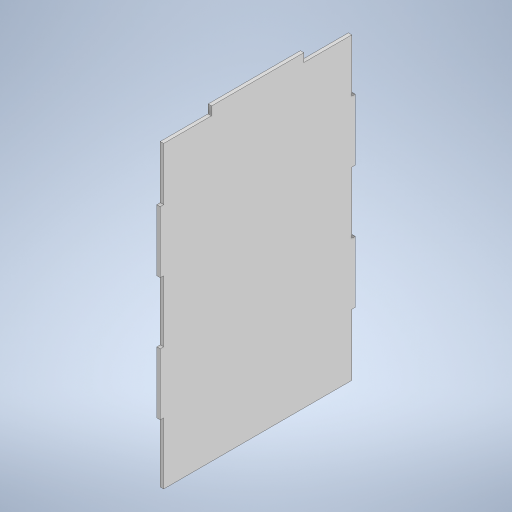
# Autodesk Inventor part: inner_side
Saved by Autodesk Inventor 2023 (Build 270158000, 158)
## iProperties
Created: 2023-04-26
Part Number: inner_side
Material: Generic
Document SubType Name: Modeling
Designer: Unnar
Density: 1 g/cm^3
Appearance: Default
Author: Unnar
Autodesk Inventor part; units mm, degrees
ref_plane "YZ Plane" through (0, 0, 0) normal (1, 0, 0) x (0, 1, 0)
ref_plane "XZ Plane" through (0, 0, 0) normal (0, 1, 0) x (-1, 0, 0)
ref_plane "XY Plane" through (0, 0, 0) normal (0, 0, 1) x (1, 0, 0)
sketch "Sketch1" plane through (0, 0, 0) normal (1, 0, 0) x (0, 1, 0)
  line L0 (66.9402, 52.2533) -> (-113.0598, 52.2533)
  line L1 (-113.0598, 52.2533) -> (-113.0598, -61.7467)
  line L2 (-113.0598, -61.7467) -> (66.9402, -61.7467)
  line L3 (66.9402, -61.7467) -> (66.9402, 52.2533)
  point P0 (0, 0)
  dimension "d0" = 114
  dimension "d1" = 180
  constraints: 8 end point, 2 parallel, 1 horizontal, 1 perpendicular
  measures "d0" distance of L2.end L0.start
  measures "d1" distance of L0.start L0.end
extrude "Extrusion1" add sketch "Sketch1" along normal blind 2
sketch "Sketch2" plane through (2, 0, 0) normal (1, 0, 0) x (0, 0, -1)
  line L0 (61.7467, 66.9402) -> (-52.2533, 66.9402) projected
  line L1 (-52.2533, 66.9402) -> (-22.2533, 66.9402)
  line L2 (-22.2533, 66.9402) -> (-22.2533, 61.9402)
  line L3 (-22.2533, 61.9402) -> (-52.2533, 61.9402)
  line L4 (-52.2533, 61.9402) -> (-52.2533, 66.9402)
  line L5 (61.7467, 66.9402) -> (31.7467, 66.9402)
  line L6 (31.7467, 66.9402) -> (31.7467, 61.9402)
  line L7 (31.7467, 61.9402) -> (61.7467, 61.9402)
  line L8 (61.7467, 61.9402) -> (61.7467, 66.9402)
  point P0 (0, 0)
  point P1 (31.7467, 66.9402)
  dimension "d4" = 30
  dimension "d5" = 30
  dimension "d6" = 5
  constraints: 16 end point, 4 parallel, 2 horizontal, 2 perpendicular, 1 point on line
  measures "d4" distance of L2.end L3.end
  measures "d5" distance of L6.end L7.end
  measures "d6" distance of L3.end L0.end
extrude "Extrusion2" cut sketch "Sketch2" against normal blind 2
sketch "Sketch3" plane through (2, 0, 0) normal (1, 0, 0) x (0, 0, -1)
  line L0 (-52.2533, 61.9402) -> (-52.2533, -113.0598) projected
  line L1 (-52.2533, -113.0598) -> (-50.2533, -113.0598)
  line L2 (-50.2533, -113.0598) -> (-50.2533, -77.0598)
  line L3 (-50.2533, -77.0598) -> (-52.2533, -77.0598)
  line L4 (-52.2533, -77.0598) -> (-52.2533, -113.0598)
  line L5 (-52.2533, -41.0598) -> (-50.2533, -41.0598)
  line L6 (-50.2533, -41.0598) -> (-50.2533, -5.0598)
  line L7 (-50.2533, -5.0598) -> (-52.2533, -5.0598)
  line L8 (-52.2533, -5.0598) -> (-52.2533, -41.0598)
  line L9 (-52.2533, 61.9402) -> (-50.2533, 61.9402)
  line L10 (-50.2533, 61.9402) -> (-50.2533, 30.9402)
  line L11 (-50.2533, 30.9402) -> (-52.2533, 30.9402)
  line L12 (-52.2533, 30.9402) -> (-52.2533, 61.9402)
  line L13 (61.7467, 61.9402) -> (31.7467, 61.9402) projected
  line L14 (61.7467, 61.9402) -> (59.7467, 61.9402)
  line L15 (59.7467, 61.9402) -> (59.7467, 30.9402)
  line L16 (59.7467, 30.9402) -> (61.7467, 30.9402)
  line L17 (61.7467, 30.9402) -> (61.7467, 61.9402)
  line L18 (61.7467, -113.0598) -> (61.7467, 61.9402) projected
  line L19 (61.7467, -5.0598) -> (59.7467, -5.0598)
  line L20 (59.7467, -5.0598) -> (59.7467, -41.0598)
  line L21 (59.7467, -41.0598) -> (61.7467, -41.0598)
  line L22 (61.7467, -41.0598) -> (61.7467, -5.0598)
  line L23 (-52.2533, -113.0598) -> (61.7467, -113.0598) projected
  line L24 (61.7467, -77.0598) -> (59.7467, -77.0598)
  line L25 (59.7467, -77.0598) -> (59.7467, -113.0598)
  line L26 (59.7467, -113.0598) -> (61.7467, -113.0598)
  line L27 (61.7467, -113.0598) -> (61.7467, -77.0598)
  point P0 (0, 0)
  point P1 (60.7467, -77.0598)
  point P2 (60.7467, -41.0598)
  point P3 (60.7467, -5.0598)
  point P4 (60.7467, 30.9402)
  point P5 (61.7467, -41.0598)
  dimension "d9" = 2
  dimension "d10" = 2
  dimension "d11" = 36
  dimension "d12" = 36
  dimension "d13" = 36
  dimension "d14" = 36
  dimension "d15" = 36
  constraints: 48 end point, 12 parallel, 12 point on line, 6 horizontal, 6 perpendicular, 4 midpoint
  measures "d9" distance of L10.end L11.end
  measures "d10" distance of L15.end L16.end
  measures "d11" distance of L1.end L2.end
  measures "d12" distance of L5.end L6.end
  measures "d13" distance of point (60.747, -77.06) point (60.747, -41.06)
  measures "d14" distance of point (60.747, -5.06) point (60.747, 30.94)
  measures "d15" distance of L19.end L20.end
extrude "Extrusion3" cut sketch "Sketch3" against normal blind 2
body "Solid1"
